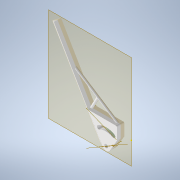
# Autodesk Inventor part: CameraArm
Saved by Autodesk Inventor 2020 (Build 240168000, 168)
## iProperties
Created: 2020-03-20
Part Number: CameraArm
Material: Generisch
Document SubType Name: Modeling
Designer: Fynn
Density: 1 g/cm^3
Appearance: Vorgabe
Author: Fynn
Autodesk Inventor part; units mm, degrees
ref_plane "YZ Plane" through (0, 0, 0) normal (1, 0, 0) x (0, 1, 0)
ref_plane "XZ Plane" through (0, 0, 0) normal (0, 1, 0) x (-1, 0, 0)
ref_plane "XY Plane" through (0, 0, 0) normal (0, 0, 1) x (1, 0, 0)
sketch "Skizze1" plane through (0, 0, 0) normal (0, 0, 1) x (1, 0, 0)
  circle A0 centre (-8.8, -6.5765) radius 1.5 projected
  circle A1 centre (-9, -18.5765) radius 1.5 projected
  line L0 (-9, -18.5765) -> (-5, -18.5765)
  line L1 (-9.0008, 0.1024) -> (5.9992, 0.1024)
  line L2 (-5, -18.5765) -> (5.9992, 0.1024)
  line L3 (-9.0008, 0.1024) -> (-24.0008, 0.1024)
  line L4 (-9, -18.5765) -> (-13, -18.5765)
  line L5 (-24.0008, 0.1024) -> (-13, -18.5765)
  arc A2 (-12.0056, -20.265) -> (-5.9977, -20.2708) centre (-9, -18.5765) ccw
  line L6 (-5, -18.5765) -> (-5.9977, -20.2708)
  line L7 (-13, -18.5765) -> (-11.9342, -20.3862)
  point P0 (0, 0)
  dimension "d1" = 4
  dimension "d2" = 15
  dimension "d3" = 15
  dimension "d5" = 4
  constraints: 16 end point, 4 horizontal, 3 point on circle, 1 centre point, 1 coincident, 1 point on line
  measures "d1" distance of L0.start L0.end
  measures "d2" distance of L1.start L1.end
  measures "d3" distance of L1.start L3.end
  measures "d5" distance of L0.start L4.end
extrude "Extrusion1" add sketch "Skizze1" along normal blind 6 contours L0 L6 A2 L7 L4 A1 | A1 L4 L5 L3 L1 L2 L0
sketch "Skizze2" plane through (0, 0, 6) normal (0, 0, 1) x (1, 0, 0)
  circle A0 centre (-9, -18.5765) radius 1.5 projected
  circle A1 centre (-8.8, -6.5765) radius 1.5 projected
  circle A2 centre (-8.8, -6.5765) radius 1.5 projected
  line L0 (-9, -18.5765) -> (-2.1491, -6.9422)
  line L1 (-5.9977, -20.2708) -> (5.9992, 0.1024) projected
  line L2 (-9, -18.5765) -> (-15.8517, -6.9427)
  line L3 (-24.0008, 0.1024) -> (-11.9342, -20.3862) projected
  line L4 (-2.1491, -6.9422) -> (-2.9102, -8.2348)
  line L5 (-15.8517, -6.9427) -> (-15.0907, -8.2348)
  arc A3 (-3.6713, -9.5272) -> (-2.1492, -6.9424) centre (-2.9102, -8.2348) ccw
  arc A4 (-15.8073, -6.9167) -> (-14.3293, -9.5276) centre (-15.0907, -8.2348) ccw
  arc A5 (-3.6713, -9.5272) -> (-14.3293, -9.5276) centre (-9, -18.5765) ccw
  arc A6 (-17.004, -11.7779) -> (-0.9964, -11.7775) centre (-9, -18.5765) ccw
  arc A7 (-2.1491, -6.9422) -> (-15.8959, -6.9689) centre (-9, -18.5765) ccw
  arc A8 (-18.5945, -9.0773) -> (0.594, -9.0767) centre (-9, -18.5765) ccw
  point P0 (0, 0)
  point P1 (-8.7514, -5.0773)
  point P2 (-8.825, -8.0763)
  point P3 (-2.1492, -6.9424)
  point P4 (-8.7986, -5.0765)
  dimension "d9" = 1.5
  constraints: 15 point on circle, 8 end point, 8 point on line, 6 centre point, 4 coincident, 2 parallel
  measures "d9" distance of L0.end L4.end
extrude "Extrusion2" cut sketch "Skizze2" against normal blind 10 contours A5 A1 A7 L0 | L0 A3 | A4 L2 | L2 A4 A7 A1 A5
sketch "Skizze3" plane through (-24.0008, 0.1024, 0) normal (0, 1, 0) x (1, 0, 0)
  line L0 (24.0008, 0) -> (24.0008, 12.6) projected
  line L1 (18.0031, -6) -> (30, -6) projected
  line L2 (24.0008, 0) -> (30, 0)
  line L3 (30, 0) -> (30, -6)
  line L4 (30, -6) -> (24.0008, -6)
  line L5 (24.0008, -6) -> (24.0008, 0)
  constraints: 8 end point, 2 parallel, 1 horizontal, 1 perpendicular
extrude "Extrusion3" cut sketch "Skizze3" against normal through all
ref_plane "Arbeitsebene1" through (-11.9342, -20.3862, 6) normal (0.5035686, -0.8639552, 0) x (0, 0, -1)
sketch "Skizze4" plane through (-11.9342, -20.3862, 6) normal (0.5035686, -0.8639552, 0) x (0, 0, -1)
  point P0 (6, 20.5765)
sketch "Skizze5" plane through (-11.9342, -20.3862, 6) normal (0.5035686, -0.8639552, 0) x (0, 0, -1)
  point P0 (6, 20.5765)
sketch "Skizze6" plane through (-11.9342, -20.3862, 6) normal (0.5035686, -0.8639552, 0) x (0, 0, -1)
  line L0 (6, 20.628) -> (6, -0.1076) projected
  line L1 (0, 20.628) -> (0, -0.1076) projected
  line L2 (6, 5.1869) -> (6, 0) projected
  line L3 (6, 0) -> (3, -5.1076)
  line L4 (3, -5.1076) -> (0, -0.1076)
  line L5 (6, -0.1076) -> (0, -0.1076) projected
  line L6 (0, -0.1076) -> (3, -0.1076)
  point P0 (6, 20.5765)
  point P1 (5.9368, -0.1076)
  dimension "d14" = 3
  dimension "d15" = 0
  dimension "d16" = 5
  constraints: 6 end point, 1 midpoint
  measures "d14" distance of L1.end L6.end
  measures "d15" horizontal distance of L3.end L6.end
  measures "d16" vertical distance of L3.end L1.end
extrude "Extrusion4" add sketch "Skizze6" against normal blind 80 contours L3 L4 L5
chamfer "Fase1" distance 2 angle 45 2 edges at (-14.1871, -21.6993, 1.5316) (-14.1871, -21.6993, 4.5)
ref_plane "Arbeitsebene2" through (-56.6324, 46.1582, 3) normal (0, 0, 1) x (1, 0, 0)
sketch "Skizze7" plane through (-56.6324, 46.1582, 3) normal (0, 0, 1) x (1, 0, 0)
  line L0 (56.6324, -46.0558) -> (56.6324, -56.2436) projected
  line L1 (56.6324, -46.0558) -> (32.6316, -46.0558) projected
  line L2 (53.6324, -46.0558) -> (20.0056, -24.3938)
  line L3 (32.6316, -46.0558) -> (4.3198, 2.5178) projected
  line L4 (20.0056, -24.3938) -> (17.1397, -22.5477)
  point P0 (56.6324, -46.1582)
  dimension "d22" = 3
  dimension "d23" = 40
  constraints: 4 end point, 2 point on line
  measures "d22" distance of L0.start L2.start
  measures "d23" distance of L2.start L2.end
sketch "Skizze8" plane through (-24.0008, 0.1024, 0) normal (0, 1, 0) x (1, 0, 0)
  line L0 (24.0008, -2.9971) -> (21.0008, -2.9971)
  circle A0 centre (21.0008, -2.9971) radius 1
  point P0 (24.0008, 0)
  dimension "d24" = 3
  dimension "d25" = 2
  constraints: 2 end point, 1 centre point, 1 coincident, 1 horizontal
  measures "d24" distance of L0.start L0.end
  measures "d25" diameter of A0
sweep "Sweeping2" add profiles "Skizze8" path "Skizze7" path curves L2 L4
sketch "Skizze9" plane through (-56.6324, 46.1582, 3) normal (0, 0, 1) x (1, 0, 0)
  line L0 (31.5707, -47.831) -> (38.0134, -35.8771)
  point P0 (56.6324, -46.1582)
  constraints: 2 end point
ref_plane "Arbeitsebene3" through (-24.0008, 0.1024, 6) normal (-0.3765595, -0.9263924, 0) x (0, 0, -1)
sketch "Skizze10" plane through (-24.0008, 0.1024, 6) normal (-0.3765595, -0.9263924, 0) x (0, 0, -1)
  line L0 (3, 14.1906) -> (3, -47.5724) projected
  circle A0 centre (3, 0.0464) radius 1
  point P0 (6, 22.2728)
  dimension "d30" = 2
  constraints: 1 centre point, 1 point on line
  measures "d30" diameter of A0
sweep "Sweeping3" add profiles "Skizze10" path "Skizze9"
fillet "Rundung1" radius 1 1 edges at (0, 0.1024, 3)
